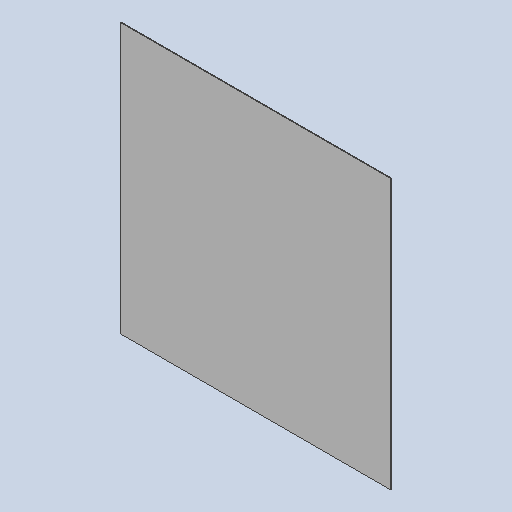
# Autodesk Inventor part: 01.1 GBK shield
Saved by Autodesk Inventor 2026.2 (Build 302298000, 298)
## iProperties
Created: 2026-04-17
Part Number: 01.1 GBK shield
Material: Steel
Document SubType Name: Sheet Metal
Designer: admin
Density: 7.85 g/cm^3
Sheet Metal Rule: Default_mm
Appearance: Default
Author: admin
Autodesk Inventor part; units mm, degrees
ref_plane "YZ Plane" through (0, 0, 0) normal (1, 0, 0) x (0, 1, 0)
ref_plane "XZ Plane" through (0, 0, 0) normal (0, 1, 0) x (-1, 0, 0)
ref_plane "XY Plane" through (0, 0, 0) normal (0, 0, 1) x (1, 0, 0)
sketch "Sketch1" plane through (0, 0, 0) normal (0, 0, 1) x (1, 0, 0)
  line L0 (745, -742.9175) -> (-745, -742.9175)
  line L1 (-745, -742.9175) -> (-745, 742.9175)
  line L2 (-745, 742.9175) -> (745, 742.9175)
  line L3 (745, 742.9175) -> (745, -742.9175)
  line L4 (745, -742.9175) -> (-745, 742.9175) construction
  line L5 (-745, -742.9175) -> (745, 742.9175) construction
  point P0 (0, 0)
  dimension "d0" = 1490
  dimension "d1" = 1485.835
  measures "d0" distance of L1.end L2.end
  measures "d1" distance of L0.end L1.end
extrude "Plate1" add sketch "Sketch1" along normal blind 4
equation "\"d0\" = высота_листа_стенки"
equation "\"d2\" = Thickness"
equation "\"BendRadius\" = Thickness"
equation "\"BendReliefWidth\" = Thickness"
equation "\"BendReliefDepth\" = 0.5 * Thickness"
equation "\"CornerReliefSize\" = 4 * Thickness"
equation "\"MinimumRemnant\" = 2 * Thickness"
equation "\"TransitionRadius\" = BendRadius"
equation "\"JacobiRadiusSize\" = BendRadius"
equation "\"GapSize\" = Thickness"
equation "\"высота_листа_стенки\" = 1490"
equation "\"Thickness\" = 4"
body "Solid1"
